# Autodesk Inventor part: piece-fixer
Saved by Autodesk Inventor 2015 (Build 190159000, 159)
## iProperties
Created: 2014-11-30
Part Number: piece-fixer
Material: Generic
Document SubType Name: Modeling
Designer: Adam
Density: 1 g/cm^3
Appearance: Default
Author: Adam
Autodesk Inventor part; units mm, degrees
ref_plane "YZ Plane" through (0, 0, 0) normal (1, 0, 0) x (0, 1, 0)
ref_plane "XZ Plane" through (0, 0, 0) normal (0, 1, 0) x (-1, 0, 0)
sketch "Sketch1" plane through (0, 0, 0) normal (0, 0, 1) x (1, 0, 0)
  arc A0 (0, 9) -> (-7.7942, 4.5) centre (0, 0) ccw projected
  arc A1 (-5.0533, 10.5526) -> (0, 9) centre (0, 18) ccw projected
  arc A2 (-5.0533, 10.5526) -> (-6.6121, 9.6526) centre (-5.6148, 9.7251) ccw projected
  arc A3 (-7.7942, 4.5) -> (-6.6121, 9.6526) centre (-15.5885, 9) ccw projected
  arc A4 (7.7942, 4.5) -> (0, 9) centre (0, 0) ccw projected
  arc A5 (6.6121, 9.6526) -> (7.7942, 4.5) centre (15.5885, 9) ccw projected
  arc A6 (6.6121, 9.6526) -> (5.0533, 10.5526) centre (5.6148, 9.7251) ccw projected
  arc A7 (0, 9) -> (5.0533, 10.5526) centre (0, 18) ccw projected
  arc A8 (7.7942, -4.5) -> (7.7942, 4.5) centre (0, 0) ccw projected
  arc A9 (11.6654, -0.9) -> (7.7942, -4.5) centre (15.5885, -9) ccw projected
  arc A10 (11.6654, -0.9) -> (11.6654, 0.9) centre (11.2296, 0) ccw projected
  arc A11 (7.7942, 4.5) -> (11.6654, 0.9) centre (15.5885, 9) ccw projected
  arc A12 (0, -9) -> (7.7942, -4.5) centre (0, 0) ccw projected
  arc A13 (5.0533, -10.5526) -> (0, -9) centre (0, -18) ccw projected
  arc A14 (5.0533, -10.5526) -> (6.6121, -9.6526) centre (5.6148, -9.7251) ccw projected
  arc A15 (7.7942, -4.5) -> (6.6121, -9.6526) centre (15.5885, -9) ccw projected
  arc A16 (-7.7942, -4.5) -> (0, -9) centre (0, 0) ccw projected
  arc A17 (-6.6121, -9.6526) -> (-7.7942, -4.5) centre (-15.5885, -9) ccw projected
  arc A18 (-6.6121, -9.6526) -> (-5.0533, -10.5526) centre (-5.6148, -9.7251) ccw projected
  arc A19 (0, -9) -> (-5.0533, -10.5526) centre (0, -18) ccw projected
  arc A20 (-7.7942, 4.5) -> (-7.7942, -4.5) centre (0, 0) ccw projected
  arc A21 (-11.6654, 0.9) -> (-7.7942, 4.5) centre (-15.5885, 9) ccw projected
  arc A22 (-11.6654, 0.9) -> (-11.6654, -0.9) centre (-11.2296, 0) ccw projected
  arc A23 (-7.7942, -4.5) -> (-11.6654, -0.9) centre (-15.5885, -9) ccw projected
  circle A24 centre (0, 0) radius 6.5
  point P0 (0, 0)
  constraints: 1 centre point, 2 other
ref_plane "Work Plane1" through (-9, -9, 1.25) normal (0, 0, 1) x (1, 0, 0)
extrude "Extrusion1" add sketch "Sketch1" along normal up to surface (1.25 mm away)
body "Solid1"
